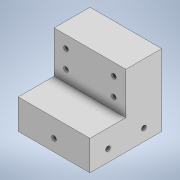
# Autodesk Inventor part: Base_V2b
Saved by Autodesk Inventor 2022 (Build 260153000, 153)
## iProperties
Created: 2022-06-15
Part Number: Base_V2b
Material: Generic
Document SubType Name: Modeling
Designer: Asus
Density: 1 g/cm^3
Appearance: Default
Author: Asus
Autodesk Inventor part; units mm, degrees
ref_plane "YZ Plane" through (0, 0, 0) normal (1, 0, 0) x (0, 1, 0)
ref_plane "XZ Plane" through (0, 0, 0) normal (0, 1, 0) x (-1, 0, 0)
ref_plane "XY Plane" through (0, 0, 0) normal (0, 0, 1) x (1, 0, 0)
sketch "Sketch1" plane through (0, 0, 0) normal (0, 0, 1) x (1, 0, 0)
  line L0 (-30, 30) -> (30, 30)
  line L1 (30, 30) -> (30, -30)
  line L2 (30, -30) -> (-30, -30)
  line L3 (-30, -30) -> (-30, 30)
  point P0 (0, 0)
  dimension "d0" = 60
  dimension "d1" = 60
  dimension "d2" = 30
  dimension "d3" = 30
  constraints: 8 end point, 2 parallel, 1 horizontal, 1 perpendicular
  measures "d0" distance of L0.end L1.end
  measures "d1" distance of L0.start L0.end
  measures "d2" distance from line of point (0, 0) L1
  measures "d3" distance from line of L0 point (0, 0)
extrude "Extrusion1" add sketch "Sketch1" along normal blind 10
sketch "Sketch2" plane through (0, 0, 10) normal (0, 0, 1) x (1, 0, 0)
  line L0 (30, 30) -> (-30, 30) projected
  line L1 (30, -30) -> (30, 30) projected
  line L2 (-30, 30) -> (30, 30)
  line L3 (30, 30) -> (30, -5)
  line L4 (30, -5) -> (-30, -5)
  line L5 (-30, -5) -> (-30, 30)
  point P0 (0, 0)
  dimension "d6" = 35
  constraints: 8 end point, 2 parallel, 1 horizontal, 1 perpendicular, 1 point on line
  measures "d6" distance between parallel lines of L0 L4
extrude "Extrusion2" add sketch "Sketch2" along normal blind 20
sketch "Sketch3" plane through (0, 0, 10) normal (0, 0, 1) x (1, 0, 0)
  line L0 (-30, -5) -> (30, -5) projected
  line L1 (-30, -30) -> (30, -30) projected
  line L2 (-30, -5) -> (30, -5)
  line L3 (30, -5) -> (30, -30)
  line L4 (30, -30) -> (-30, -30)
  line L5 (-30, -30) -> (-30, -5)
  point P0 (0, 0)
  constraints: 8 end point, 2 parallel, 1 horizontal, 1 perpendicular
extrude "Extrusion3" add sketch "Sketch3" along normal blind 50
sketch "Sketch4" plane through (0, 0, 0) normal (0, 0, -1) x (-1, 0, 0)
  circle A0 centre (-20, 20) radius 1.95
  circle A1 centre (20, 20) radius 1.95
  circle A2 centre (20, 5) radius 1.95
  circle A3 centre (-20, 5) radius 1.95
  line L0 (-30, 30) -> (30, 30) projected
  line L1 (-30, -30) -> (-30, 30) projected
  line L2 (30, 30) -> (30, -30) projected
  point P0 (0, 0)
  dimension "d11" = 10
  dimension "d12" = 10
  dimension "d13" = 10
  dimension "d14" = 10
  dimension "d15" = 10
  dimension "d16" = 25
  dimension "d17" = 25
  dimension "d18" = 10
  dimension "d19" = 3.9
  dimension "d20" = 3.9
  dimension "d21" = 3.9
  dimension "d22" = 3.9
  constraints: 4 centre point
  measures "d11" distance from line of L0 A0.centre
  measures "d12" distance from line of L1 A0.centre
  measures "d13" distance from line of L0 A1.centre
  measures "d14" distance from line of L2 A1.centre
  measures "d15" distance from line of L2 A2.centre
  measures "d16" distance from line of L0 A2.centre
  measures "d17" distance from line of L0 A3.centre
  measures "d18" distance from line of L1 A3.centre
  measures "d19" diameter of A0
  measures "d20" diameter of A1
  measures "d21" diameter of A3
  measures "d22" diameter of A2
extrude "Extrusion4" cut sketch "Sketch4" against normal blind 30
sketch "Sketch5" plane through (0, 0, 0) normal (0, 0, -1) x (-1, 0, 0)
  circle A0 centre (-20, 20) radius 1.95 projected
  circle A1 centre (-20, 20) radius 4.5
  circle A2 centre (-20, 5) radius 1.95 projected
  circle A3 centre (-20, 5) radius 4.5
  circle A4 centre (20, 20) radius 1.95 projected
  circle A5 centre (20, 20) radius 4.5
  circle A6 centre (20, 5) radius 1.95 projected
  circle A7 centre (20, 5) radius 4.5
  point P0 (0, 0)
  dimension "d25" = 9
  dimension "d26" = 9
  dimension "d27" = 9
  dimension "d28" = 9
  constraints: 4 centre point, 4 coincident
  measures "d25" diameter of A1
  measures "d26" diameter of A3
  measures "d27" diameter of A5
  measures "d28" diameter of A7
extrude "Extrusion5" cut sketch "Sketch5" against normal blind 20
sketch "Sketch6" plane through (-30, -30, 0) normal (-1, 0, 0) x (0, 0, 1)
  circle A0 centre (15, 10) radius 1.95
  circle A1 centre (45, 10) radius 1.95
  line L0 (0, 60) -> (0, 0) projected
  line L1 (0, 0) -> (60, 0) projected
  line L2 (60, 25) -> (60, 0) projected
  point P0 (0, 30)
  dimension "d31" = 15
  dimension "d32" = 10
  dimension "d33" = 15
  dimension "d34" = 10
  dimension "d35" = 3.9
  dimension "d36" = 3.9
  constraints: 2 centre point
  measures "d31" distance from line of L0 A0.centre
  measures "d32" distance from line of L1 A0.centre
  measures "d33" distance from line of L2 A1.centre
  measures "d34" distance from line of L1 A1.centre
  measures "d35" diameter of A0
  measures "d36" diameter of A1
extrude "Extrusion6" cut sketch "Sketch6" against normal blind 15
sketch "Sketch7" plane through (30, -30, 0) normal (1, 0, 0) x (0, 0, -1)
  circle A0 centre (-45, 10) radius 1.95 projected
  circle A1 centre (-45, 10) radius 1.95
  circle A2 centre (-15, 10) radius 1.95 projected
  circle A3 centre (-15, 10) radius 1.95
  point P0 (0, 30)
  constraints: 2 centre point, 2 coincident
extrude "Extrusion7" cut sketch "Sketch7" against normal blind 15
sketch "Sketch8" plane through (0, 0, 0) normal (0, 0, -1) x (-1, 0, 0)
  circle A0 centre (0, -20) radius 1.95
  line L0 (30, -30) -> (-30, -30) projected
  line L1 (-30, -30) -> (-30, 30) projected
  point P0 (0, 0)
  dimension "d41" = 10
  dimension "d42" = 30
  dimension "d43" = 3.9
  constraints: 1 centre point
  measures "d41" distance from line of L0 A0.centre
  measures "d42" distance from line of L1 A0.centre
  measures "d43" diameter of A0
extrude "Extrusion8" cut sketch "Sketch8" against normal blind 15
sketch "Sketch9" plane through (0, 0, 60) normal (0, 0, 1) x (1, 0, 0)
  circle A0 centre (0, -20) radius 1.95 projected
  circle A1 centre (0, -20) radius 1.95
  point P0 (0, 0)
  constraints: 1 centre point, 1 coincident
extrude "Extrusion9" cut sketch "Sketch9" against normal blind 15
body "Solid1"
